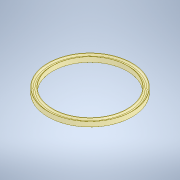
# Autodesk Inventor part: 201555-1-1-test
Saved by Autodesk Inventor 2021 (Build 250183000, 183)
## iProperties
Created: 2020-06-29
Part Number: 201555-1-1-test
Material: Nylon 6/6
Document SubType Name: Modeling
Density: 1.13 g/cm^3
Appearance: Nylon 6
Mass: 19.7025 g
Surface Area: 104.615 cm^2
Volume: 17.4358 cm^3
Author: MK
Subject: 100/120*5
Autodesk Inventor part; units mm, degrees
ref_plane "YZ Plane" through (0, 0, 0) normal (1, 0, 0) x (0, 1, 0)
ref_plane "XZ Plane" through (0, 0, 0) normal (0, 1, 0) x (-1, 0, 0)
ref_plane "XY Plane" through (0, 0, 0) normal (0, 0, 1) x (1, 0, 0)
sketch "Sketch1" plane through (0, 0, 0) normal (0, 0, 1) x (1, 0, 0)
  line L0 (129.8, 7.5) -> (129.8, -7.5)
  line L1 (129.8, -7.5) -> (115.2, -7.5)
  line L2 (115.2, -7.5) -> (115.2, 7.5)
  line L3 (0, 7.1027) -> (0, -7.1027)
  line L4 (116.2607, 7.0607) -> (120.3787, 2.9426)
  line L5 (128.7393, 7.0607) -> (124.6213, 2.9426)
  arc A0 (120.3787, 2.9426) -> (124.6213, 2.9426) centre (122.5, 5.064) ccw
  arc A1 (129.8, 7.5) -> (128.7393, 7.0607) centre (129.8, 6) ccw
  line L6 (122.5, 5.064) -> (122.5, 12.2512)
  arc A2 (116.2607, 7.0607) -> (115.2, 7.5) centre (115.2, 6) ccw
  point P0 (0, 0)
  point P1 (0, 0)
  point P2 (115.2, 0)
  point P3 (129.8, -3.0792)
  point P4 (115.2, 0)
  dimension "externalDiameter_parameter" = 259.6
  dimension "d5" = 230.4
  dimension "d1" = 90
  dimension "fascia_parameter" = 14.6
  dimension "radius1_parameter" = 1.5
  dimension "radius2_parameter" = 3
  dimension "d2" = 90
  dimension "height_parameter" = 15
  dimension "d28" = 1.5
  constraints: 14 end point, 6 point on circle, 4 tangent, 3 centre point, 3 midpoint, 2 coincident, 2 horizontal alignment, 2 vertical, 2 vertical alignment, 1 parallel, 1 point on line, 1 symmetric about line, 1 other
  measures "externalDiameter_parameter" diameter of L0 L3
  measures "d5" diameter of L2 L3
  measures "d1" angle of L5 L4
  measures "fascia_parameter" distance between parallel lines of L0 L2
  measures "radius1_parameter" radius of A1
  measures "radius2_parameter" radius of A0
  measures "d2" angle of L1 L2
  measures "height_parameter" distance from line of L1 L0.start
  measures "d28" radius of A2
revolve "Revolution2" add sketch "Sketch1" angle 360 about axis through (0, 7.1027, 0) along (0, -1, 0)
fillet "Fillet2" radius 0.3 2 edges at (-129.8, -7.5, 0) (-115.2, -7.5, 0)
body "Solid2"
